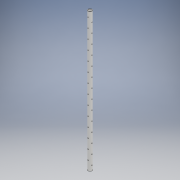
# Autodesk Inventor part: Ground_Antenna700mm_Support
Saved by Autodesk Inventor 2018 (Build 220112000, 112)
## iProperties
Created: 2018-10-12
Part Number: Ground_Antenna700mm_Support
Material: PVC-Piping
Document SubType Name: Modeling
Designer: Bradley
Density: 1.4 g/cm^3
Appearance: Smooth - White
Mass: 594.901 g
Surface Area: 2131.77 cm^2
Volume: 424.929 cm^3
Author: Bradley
Autodesk Inventor part; units mm, degrees
ref_plane "YZ Plane" through (0, 0, 0) normal (1, 0, 0) x (0, 1, 0)
ref_plane "XZ Plane" through (0, 0, 0) normal (0, 1, 0) x (-1, 0, 0)
ref_plane "XY Plane" through (0, 0, 0) normal (0, 0, 1) x (1, 0, 0)
sketch "Sketch1" plane through (0, 0, 0) normal (0, 0, 1) x (1, 0, 0)
  circle A0 centre (0, 0) radius 16.7005
  circle A1 centre (0, 0) radius 12.7
  dimension "d0" = 33.401
  dimension "d1" = 25.4
  constraints: 2 centre point, 2 coincident
  measures "d0" diameter of A0
  measures "d1" diameter of A1
extrude "Extrusion1" add sketch "Sketch1" along normal mid plane 1150
sketch "Sketch3" plane through (0, 0, 0) normal (1, 0, 0) x (0, 1, 0)
  line L0 (-16.7005, -575) -> (-16.7005, 575) projected
  line L1 (12.7, -575) -> (-12.7, -575) projected
  point P0 (0, 0)
  point P1 (0, -534.236)
  point P2 (0, -575)
  point P3 (0, -454.936)
  point P4 (0, -375.636)
  point P5 (0, -296.336)
  point P6 (0, -217.036)
  point P7 (0, -137.736)
  point P8 (0, -58.436)
  point P9 (0, 20.864)
  point P10 (0, 100.164)
  point P11 (0, 179.464)
  point P12 (0, 258.764)
  point P13 (0, 338.064)
  point P14 (0, 417.364)
  point P15 (0, 496.664)
  dimension "d19" = 40.764
  dimension "d22" = 79.3
  constraints: 1 midpoint, 1 vertical, 1 vertical alignment, 13 other
  measures "d19" distance from line of L1 point (0, -534.236)
  measures "d22" distance of point (0, -534.236) point (0, -454.936)
hole "Hole2" at (0, 0, -534.236) at (0, 0, -454.936) at (0, 0, -375.636) at (0, 0, -296.336) at (0, 0, -217.036) at (0, 0, -137.736) at (0, 0, -58.436) at (0, 0, 20.864) at (0, 0, 100.164) at (0, 0, 179.464) at (0, 0, 258.764) at (0, 0, 338.064) at (0, 0, 417.364) at (0, 0, 496.664) direction (-1, 0, 0) diameter 6.35 end through all both
sketch "Sketch4" plane through (0, 0, 0) normal (0, 1, 0) x (-1, 0, 0)
  line L0 (16.7005, -537.411) -> (12.7, -537.411) projected
  line L1 (-12.7, -458.111) -> (-16.7005, -458.111) projected
  line L2 (-12.7, -458.111) -> (12.7, -537.411) construction
  line L3 (-16.7005, -575) -> (-16.7005, 575) projected
  point P0 (0, 0)
  point P1 (0, -497.761)
  point P2 (0, -418.461)
  point P3 (0, -339.161)
  point P4 (0, -259.861)
  point P5 (0, -180.561)
  point P6 (0, -101.261)
  point P7 (0, -21.961)
  point P8 (0, 57.339)
  point P9 (0, 136.639)
  point P10 (0, 215.939)
  point P11 (0, 295.239)
  point P12 (0, 374.539)
  point P13 (0, 453.839)
  point P14 (0, 533.139)
  dimension "d36" = 79.3
  constraints: 2 end point, 1 midpoint, 1 vertical, 13 other
  measures "d36" distance of point (0, -497.761) point (0, -418.461)
hole "Hole3" at (0, 0, -497.761) at (0, 0, -418.461) at (0, 0, -339.161) at (0, 0, -259.861) at (0, 0, -180.561) at (0, 0, -101.261) at (0, 0, -21.961) at (0, 0, 57.339) at (0, 0, 136.639) at (0, 0, 215.939) at (0, 0, 295.239) at (0, 0, 374.539) at (0, 0, 453.839) at (0, 0, 533.139) direction (0, -1, 0) diameter 6.35 end through all both
equation "\"d36\" = d22"
body "Solid1"
